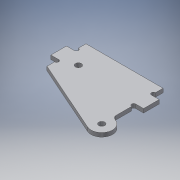
# Autodesk Inventor part: 付け根_サブフレーム_6_1
Saved by Autodesk Inventor 2018 (Build 220112000, 112)
## iProperties
Created: 2016-08-24
Part Number: 付け根_サブフレーム_6_1
Material: アルミニウム 2014-T4
Document SubType Name: Modeling
Designer: hiro
Density: 2.8 g/cm^3
Appearance: サテン
Mass: 4.80467 g
Surface Area: 23.01 cm^2
Volume: 1.71595 cm^3
Author: hiro
Autodesk Inventor part; units mm, degrees
ref_plane "YZ Plane" through (0, 0, 0) normal (1, 0, 0) x (0, 1, 0)
ref_plane "XZ Plane" through (0, 0, 0) normal (0, 1, 0) x (-1, 0, 0)
ref_plane "XY Plane" through (0, 0, 0) normal (0, 0, 1) x (1, 0, 0)
sketch "スケッチ1" plane through (0, 0, 0) normal (0, 0, 1) x (1, 0, 0)
  circle A0 centre (-16, 10) radius 1.55
  circle A1 centre (16, -10) radius 1.55
  line L0 (-16, 10) -> (16, -10) construction
  line L1 (-23.6, 38) -> (15.9, 38) construction
  line L2 (15.9, 38) -> (15.9, -13.5) construction
  line L3 (15.9, -13.5) -> (-23.6, -13.5) construction
  line L4 (-23.6, -13.5) -> (-23.6, 38) construction
  line L5 (-23.6, 10) -> (15.9, 10) construction
  line L6 (15.9, 15.5) -> (19.9, 15.5)
  line L7 (19.9, 15.5) -> (19.9, 7.5)
  line L8 (19.9, 7.5) -> (15.9, 7.5)
  line L9 (-23.6, 15.5) -> (-27.6, 15.5)
  line L10 (-27.6, 15.5) -> (-27.6, 7.5)
  line L11 (-27.6, 7.5) -> (-23.6, 7.5)
  line L12 (-23.6, 17.6) -> (-23.6, 21.5)
  line L13 (-23.6, 21.5) -> (15.9, 21.5)
  line L14 (15.9, 21.5) -> (15.9, 17.6)
  circle A2 centre (16, -10) radius 5.5 construction
  arc A3 (-23.6, 15.5) -> (-23.6, 17.6) centre (-23.6, 16.55) ccw
  arc A4 (15.9, 17.6) -> (15.9, 15.5) centre (15.9, 16.55) ccw
  arc A5 (-23.6, 5.4) -> (-23.6, 7.5) centre (-23.6, 6.45) ccw
  line L15 (-23.6, 5.4) -> (-23.6, 1.5)
  line L16 (-23.6, 1.5) -> (13.7754, -15.03)
  arc A6 (15.9, 7.5) -> (15.9, 5.4) centre (15.9, 6.45) ccw
  line L17 (15.9, 5.4) -> (15.9, -4)
  line L18 (15.9, -4) -> (18.1154, -4.9231)
  arc A7 (13.7754, -15.03) -> (18.1154, -4.9231) centre (16, -10) ccw
  circle A8 centre (-16, 10) radius 5.6 construction
  circle A9 centre (-16, 10) radius 7.6 construction
  line L19 (16, -6.5359) -> (19, -8.2679) construction
  line L20 (19, -8.2679) -> (19, -11.7321) construction
  line L21 (19, -11.7321) -> (16, -13.4641) construction
  line L22 (16, -13.4641) -> (13, -11.7321) construction
  line L23 (13, -11.7321) -> (13, -8.2679) construction
  line L24 (13, -8.2679) -> (16, -6.5359) construction
  circle A10 centre (-16, 10) radius 8.25 construction
  circle A11 centre (-16, 18.25) radius 1.55
  circle A12 centre (-24.25, 10) radius 1.55
  circle A13 centre (-16, 1.75) radius 1.55
  circle A14 centre (-7.75, 10) radius 1.55
  point P0 (0, 0)
  point P1 (0, 0)
  point P2 (-27.6, 11.5)
  point P3 (19.9, 11.5)
  dimension "d76" = 16.5
  dimension "d37" = 20
  dimension "d47" = 32
  dimension "d48" = 3.1
  dimension "d49" = 51.5
  dimension "d50" = 39.5
  dimension "d51" = 28
  dimension "d52" = 8
  dimension "d53" = 4
  dimension "d54" = 26.5
  dimension "d56" = 1.05
  dimension "d57" = 6
  dimension "d58" = 11.2
  dimension "d59" = 2
  dimension "d64" = 3.1
  dimension "d65" = 6
  dimension "d66" = 11
  dimension "d75" = 3.1
  dimension "d79" = 360
  dimension "d85" = 6
  constraints: 50 end point, 14 centre point, 12 point on line, 10 point on circle, 8 perpendicular, 6 coincident, 5 tangent, 4 equal length, 3 equal radius, 3 horizontal, 3 midpoint, 2 collinear, 2 horizontal alignment, 2 parallel, 2 vertical, 2 vertical alignment, 24 other
  measures "d37" vertical distance of L0.end L0.start
  measures "d47" horizontal distance of L0.end L0.start
  measures "d48" diameter of A0
  measures "d49" distance of L1.end L2.end
  measures "d50" distance of L1.start L1.end
  measures "d51" distance between parallel lines of L5 L1
  measures "d52" distance of L6.end L7.end
  measures "d53" distance of L6.start L6.end
  measures "d54" distance from line of L1 point (19.9, 11.5)
  measures "d56" radius of A3
  measures "d57" distance between parallel lines of L9 L13
  measures "d58" diameter of A8
  measures "d59" radial gap between concentric circles of A9 A8
  measures "d64" diameter of A1
  measures "d65" distance between parallel lines of L20 L23
  measures "d66" diameter of A2
  measures "d75" diameter of A11
  measures "d85" vertical distance of L0.end L17.end
extrude "押し出し1" add sketch "スケッチ1" along normal blind 2 contours L6 L7 L8 A6 L17 L18 A7 L16 L15 A5 L11 L10 L9 A3 L12 L13 L14 A4 | A12
fillet "フィレット1" radius 2 1 edges at (15.9, -4, 1)
sketch "スケッチ4" plane through (0, 0, 0) normal (0, 0, -1) x (-1, 0, 0)
  circle A0 centre (16, 18.25) radius 1.55 projected
  circle A1 centre (16, 18.25) radius 1.55
  circle A2 centre (7.75, 10) radius 1.55 projected
  circle A3 centre (7.75, 10) radius 1.55
  circle A4 centre (16, 1.75) radius 1.55 projected
  circle A5 centre (16, 1.75) radius 1.55
  point P0 (0, 0)
  constraints: 3 centre point, 3 coincident
extrude "押し出し4" add sketch "スケッチ4" against normal up to surface (2 mm away)
equation "\"d37\" = d6"
equation "\"d47\" = d5"
equation "\"d52\" = d46"
equation "\"d6\" = 20"
equation "\"d5\" = 32"
equation "\"d46\" = 8"
